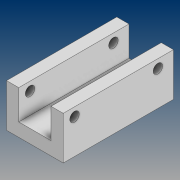
# Autodesk Inventor part: Part5
Saved by Autodesk Inventor 2021 (Build 250183000, 183)
## iProperties
Created: 2024-04-05
Part Number: Part5
Material: Generic
Document SubType Name: Modeling
Designer: Admin
Density: 1 g/cm^3
Appearance: Default
Author: Admin
Autodesk Inventor part; units mm, degrees
ref_plane "YZ Plane" through (0, 0, 0) normal (1, 0, 0) x (0, 1, 0)
ref_plane "XZ Plane" through (0, 0, 0) normal (0, 1, 0) x (-1, 0, 0)
ref_plane "XY Plane" through (0, 0, 0) normal (0, 0, 1) x (1, 0, 0)
sketch "Sketch1" plane through (0, 0, 0) normal (0, 1, 0) x (-1, 0, 0)
  line L0 (-9.5451, 18.566) -> (9.5451, 18.566)
  line L1 (9.5451, 18.566) -> (9.5451, -18.566)
  line L2 (9.5451, -18.566) -> (-9.5451, -18.566)
  line L3 (-9.5451, -18.566) -> (-9.5451, 18.566)
  line L4 (-9.5451, 18.566) -> (9.5451, -18.566) construction
  line L5 (9.5451, 18.566) -> (-9.5451, -18.566) construction
  line L6 (-5.4388, 18.566) -> (5.4388, 18.566)
  line L7 (5.4388, 18.566) -> (5.4388, -18.566)
  line L8 (5.4388, -18.566) -> (-5.4388, -18.566)
  line L9 (-5.4388, -18.566) -> (-5.4388, 18.566)
  line L10 (-5.4388, 18.566) -> (5.4388, -18.566) construction
  line L11 (5.4388, 18.566) -> (-5.4388, -18.566) construction
  point P0 (0, 0)
  constraints: 24 end point, 4 midpoint, 4 parallel, 2 horizontal, 2 perpendicular, 1 point on line
extrude "Extrusion1" add sketch "Sketch1" along normal blind 10 contours L0 L9 L2 L3 | L0 L1 L2 L7
extrude "Extrusion2" add sketch "Sketch1" against normal blind 4.5
sketch "Sketch2" plane through (9.5451, 10, 18.566) normal (1, 0, 0) x (0, 0, -1)
  line L0 (3.8006, -2.9012) -> (31.8899, -2.9012)
  point P0 (18.566, -10)
  constraints: 2 end point, 1 horizontal
hole "Hole1" at (9.5451, 7.0988, 14.7655) at (9.5451, 7.0988, -13.3239) direction (-1, 0, 0) diameter 3.2 end through all
body "Solid1"
